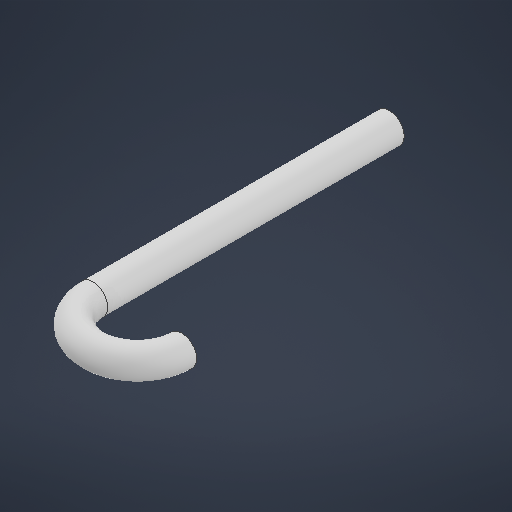
# Autodesk Inventor part: lampa
Saved by Autodesk Inventor 2026.2 (Build 302298000, 298)
## iProperties
Created: 2025-11-29
Part Number: lampa
Material: Generic
Document SubType Name: Modeling
Designer: piotr
Density: 1 g/cm^3
Appearance: Default
Author: piotr
Autodesk Inventor part; units mm, degrees
ref_plane "YZ Plane" through (0, 0, 0) normal (1, 0, 0) x (0, 1, 0)
ref_plane "XZ Plane" through (0, 0, 0) normal (0, 1, 0) x (-1, 0, 0)
ref_plane "XY Plane" through (0, 0, 0) normal (0, 0, 1) x (1, 0, 0)
sketch "Sketch15" plane through (0, 0, 0) normal (0, 0, 1) x (1, 0, 0)
  circle A0 centre (0, 0) radius 5
  circle A1 centre (0, 0) radius 4
  line L0 (-5, 5.5558) -> (-5, -5.9094)
  line L1 (-5, 5.5558) -> (-12.7265, 5.5558)
  line L2 (-12.7265, 5.5558) -> (-12.7265, -5.9094)
  line L3 (-12.7265, -5.9094) -> (-5, -5.9094)
  line L4 (-5, -5.9094) -> (-5, 5.5558)
  dimension "d48" = 10
  dimension "d49" = 8
  constraints: 10 end point, 2 centre point, 2 coincident, 2 parallel, 1 horizontal, 1 perpendicular, 1 tangent, 1 vertical
  measures "d48" diameter of A0
  measures "d49" diameter of A1
extrude "Extrusion3" add sketch "Sketch15" along normal blind 100 contours A0
sketch "Sketch16" plane through (0, 0, 100) normal (0, 0, 1) x (1, 0, 0)
  circle A0 centre (0, 0) radius 5
  circle A1 centre (0, 0) radius 4
  line L0 (15, -5) -> (15, 5)
  constraints: 2 centre point, 2 coincident, 2 end point, 1 vertical
revolve "Revolution2" add sketch "Sketch16" angle 180 about axis through (15, -5, 100) along (0, 1, 0)
body "Solid3"
